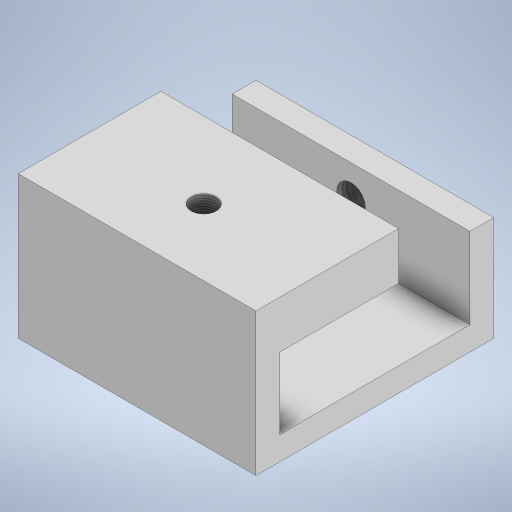
# Autodesk Inventor part: Chasis Depan Roda Kiri
Saved by Autodesk Inventor 2023 (Build 270158000, 158)
## iProperties
Created: 2025-05-21
Part Number: Chasis Depan Roda Kiri
Material: Generic
Document SubType Name: Modeling
Designer: ASUS
Density: 1 g/cm^3
Appearance: Default
Author: ASUS
Autodesk Inventor part; units mm, degrees
ref_plane "YZ Plane" through (0, 0, 0) normal (1, 0, 0) x (0, 1, 0)
ref_plane "XZ Plane" through (0, 0, 0) normal (0, 1, 0) x (-1, 0, 0)
ref_plane "XY Plane" through (0, 0, 0) normal (0, 0, 1) x (1, 0, 0)
sketch "Sketch1" plane through (0, 0, 0) normal (0, 0, 1) x (1, 0, 0)
  line L0 (48.2273, 127.3576) -> (98.2273, 127.3576)
  line L1 (98.2273, 127.3576) -> (98.2273, 105.3576)
  line L2 (98.2273, 105.3576) -> (48.2273, 105.3576)
  line L3 (48.2273, 105.3576) -> (48.2273, 127.3576)
  point P0 (0, 0)
  dimension "d8" = 50
  dimension "d9" = 22
  constraints: 8 end point, 2 parallel, 1 horizontal, 1 perpendicular
  measures "d8" distance of L1.end L2.end
  measures "d9" distance of L0.end L1.end
extrude "Extrusion1" add sketch "Sketch1" along normal blind 5
sketch "Sketch2" plane through (98.2273, 105.3576, 0) normal (1, 0, 0) x (0, 0, -1)
  line L0 (-5, 0) -> (-50, 0)
  line L1 (-50, 0) -> (-50, 30)
  line L2 (-50, 30) -> (-20, 30)
  line L3 (-20, 30) -> (-20, 20)
  line L4 (-20, 20) -> (-45, 20)
  line L5 (-45, 20) -> (-45, 5)
  line L6 (-45, 5) -> (-5, 5)
  line L7 (-5, 0) -> (-5, 22) projected
  line L8 (-5, 5) -> (-5, 0)
  point P0 (0, -105.3576)
  dimension "d12" = 45
  dimension "d13" = 30
  dimension "d14" = 30
  dimension "d15" = 10
  dimension "d16" = 25
  dimension "d17" = 15
  dimension "d18" = 40
  dimension "d19" = 5
  constraints: 16 end point, 3 perpendicular, 2 vertical, 1 collinear, 1 horizontal, 1 point on line
  measures "d12" distance of L0.start L0.end
  measures "d13" distance of L0.end L1.end
  measures "d14" distance of L1.end L2.end
  measures "d15" distance of L2.end L3.end
  measures "d16" distance of L3.end L4.end
  measures "d17" distance of L4.end L5.end
  measures "d18" distance of L5.end L6.end
  measures "d19" distance of L6.end L0.start
extrude "Extrusion2" add sketch "Sketch2" against normal blind 50
sketch "Sketch4" plane through (48.2273, 105.3576, 0) normal (0, -1, 0) x (1, 0, 0)
  line L0 (50, 50) -> (0, 50) projected
  circle A0 centre (25, 36) radius 2.65
  point P0 (-48.2273, 0)
  dimension "d24" = 5.3
  constraints: 1 centre point
  measures "d24" diameter of A0
extrude "Extrusion3" cut sketch "Sketch4" against normal blind 50
thread "Thread1" size "M5.5x0.5" class "6H" standard "ANSI Metric M Profile" length 43.6
thread "Thread2" size "M5.5x0.5" class "6H" standard "ANSI Metric M Profile" length 43.6
sketch "Sketch5" plane through (0, 0, 0) normal (0, 0, -1) x (-1, 0, 0)
  line L0 (-98.2273, 127.3576) -> (-48.2273, 127.3576) projected
  circle A0 centre (-73.2273, 120.7376) radius 3
  point P0 (0, 0)
  dimension "d32" = 6
  constraints: 1 centre point
  measures "d32" diameter of A0
extrude "Extrusion4" cut sketch "Sketch5" against normal blind 20
thread "Thread3" size "M6x1" class "6H" standard "ANSI Metric M Profile" length 43.6
body "Solid1"
